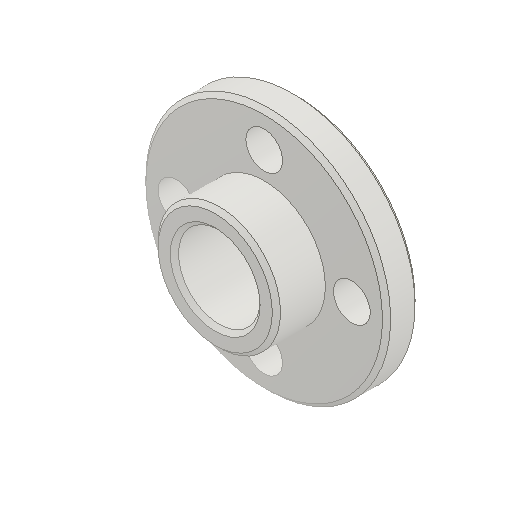
# Autodesk Inventor part: Compensador Limitador
Saved by Autodesk Inventor 2026.1 (Build 301233020, 233B)
## iProperties
Company: Elgin
Created: 2025-10-02
Part Number: Compensador Limitador
Material: Aço SAE 1045
Document SubType Name: Modeling
Designer: Willian Pinheiro
Mass: 22.0638 g
Surface Area: 22.4175 cm^2
Volume: 2.81068 cm^3
Density: 7.85 g/cm^3
Appearance: Aço
Description: Compensador Limitador
Dimensões: Ø30 x 10 mm
Total: 4
Author: Willian Pinheiro
Title: Testador Controle
Revision Number: 00
Autodesk Inventor part; units mm, degrees
ref_plane "YZ Plane" through (0, 0, 0) normal (1, 0, 0) x (0, 1, 0)
ref_plane "XZ Plane" through (0, 0, 0) normal (0, 1, 0) x (-1, 0, 0)
ref_plane "XY Plane" through (0, 0, 0) normal (0, 0, 1) x (1, 0, 0)
sketch "Esboço1" plane through (0, 0, 0) normal (0, 0, 1) x (1, 0, 0)
  line L0 (-18, 0) -> (3, 0) construction
  line L1 (0, -8) -> (0, 6) construction
  line L2 (-5, 4) -> (-5, -6)
  line L3 (-5, -6) -> (-7.5, -6)
  line L4 (-7.5, -6) -> (-7.5, 0)
  line L5 (-7.5, 0) -> (-15, 0)
  line L6 (-15, 0) -> (-15, 4)
  line L7 (-15, 4) -> (-5, 4)
  point P0 (0, 0)
  dimension "d0" = 30
  dimension "d1" = 10
  dimension "d2" = 4
  dimension "d3" = 10
  dimension "d4" = 15
  constraints: 12 end point, 5 perpendicular, 1 collinear, 1 vertical
  measures "d0" diameter of L6 L1
  measures "d1" diameter of L2 L1
  measures "d2" distance between parallel lines of L0 L7
  measures "d3" distance between parallel lines of L3 L7
  measures "d4" diameter of L4 L1
revolve "Revolução1" add sketch "Esboço1" angle 360 about axis through (0, -10, 0) along (0, 1, 0)
sketch "Esboço2" plane through (0, 4, 0) normal (0, 1, 0) x (1, 0, 0)
  line L0 (-21, 0) -> (21, 0) construction
  line L1 (0, 21) -> (0, -21) construction
  circle A0 centre (0, 0) radius 10.75 construction
  circle A1 centre (0, -10.75) radius 3.5
  circle A2 centre (0, -10.75) radius 2.25
  point P0 (-10.75, 0)
  point P1 (10.75, 0)
  point P2 (0, 10.75)
  dimension "d6" = 21.5
  dimension "d7" = 7
  dimension "d8" = 4.5
  constraints: 4 point on circle, 4 point on line, 3 centre point, 3 coincident
  measures "d6" distance of point (0, 10.75) point (0, -10.75)
  measures "d7" diameter of A1
  measures "d8" diameter of A2
hole "Furo1" at (-10.75, 4, 0) at (10.75, 4, 0) at (0, 4, 10.75) at (0, 4, -10.75) direction (0, -1, 0) diameter 4.5 end through all clearance for "Socket Head Cap Screw ISO 4762" size "M4" standard "ISO"
chamfer "Chanfro1" distance 0.5 angle 45 5 edges at (15, 4, 0) (15, 0, 0) (5, 4, 0) (5, -6, 0) (7.5, -6, 0)
